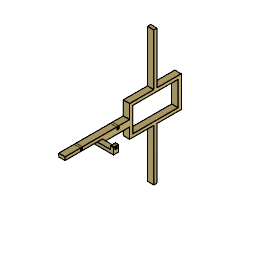
Cadru_Culisant (Autodesk Fusion 360 design; units mm, degrees)
part number: 2026-06-01-23-46-25-790
Autodesk Fusion 360 part; units mm, degrees
sketch "cadru" plane through (0, 0, 0) normal (1, 0, 0) x (0, 1, 0)
  line L0 (-20, -13.4697) -> (-20, 10.5303)
  line L1 (-17.5, -10.9697) -> (-17.5, 8.0303)
  line L2 (17.5, -10.9697) -> (-17.5, -10.9697)
  line L3 (20, -13.4697) -> (-20, -13.4697)
  line L4 (17.5, 8.0303) -> (17.5, -10.9697)
  line L5 (20, 10.5303) -> (20, -13.4697)
  line L6 (-20, 10.5303) -> (20, 10.5303)
  line L7 (-17.5, 8.0303) -> (17.5, 8.0303)
  line L8 (-1.25, 10.5303) -> (-1.25, 50.5303)
  line L9 (0, 0) -> (0, 50) construction
  line L10 (1.25, 10.5303) -> (1.25, 50.5303)
  line L11 (-1.25, 50.5303) -> (1.25, 50.5303)
  line L12 (17.5, -1.4697) -> (0, -1.4697) construction
  line L13 (-1.25, -53.4697) -> (1.25, -53.4697)
  line L14 (-1.25, -13.4697) -> (-1.25, -53.4697)
  line L15 (1.25, -13.4697) -> (1.25, -53.4697)
  line L16 (-20, -0.2197) -> (-70, -0.2197)
  line L17 (-70, -0.2197) -> (-70, -2.7197)
  line L18 (-70, -2.7197) -> (-20, -2.7197)
  line L19 (0, -1.4697) -> (-28.916, -1.4697) construction
  line L20 (-28.916, -1.4697) -> (-57.085, -1.4697) construction
  line L21 (-56.31, -0.6947) -> (-57.86, -0.6947)
  line L22 (-57.86, -0.6947) -> (-57.86, -2.2447)
  line L23 (-57.86, -2.2447) -> (-56.31, -2.2447)
  line L24 (-56.31, -2.2447) -> (-56.31, -0.6947)
  line L25 (-56.31, -0.6947) -> (-57.86, -2.2447) construction
  line L26 (-57.86, -0.6947) -> (-56.31, -2.2447) construction
  line L27 (-43.0005, -1.4697) -> (-43.0005, -15) construction
  line L28 (-45.0005, -5.2197) -> (-20, -5.2197)
  line L29 (-45.0005, -5.2197) -> (-45.0005, -0.2197)
  line L30 (-41.0005, -0.2197) -> (-41.0005, -5.2197)
  line L31 (-42.2255, -0.6947) -> (-43.7755, -0.6947)
  line L32 (-43.7755, -0.6947) -> (-43.7755, -2.2447)
  line L33 (-43.7755, -2.2447) -> (-42.2255, -2.2447)
  line L34 (-42.2255, -2.2447) -> (-42.2255, -0.6947)
  line L35 (-42.2255, -0.6947) -> (-43.7755, -2.2447) construction
  line L36 (-43.7755, -0.6947) -> (-42.2255, -2.2447) construction
  line L37 (-28.141, -0.6947) -> (-29.691, -0.6947)
  line L38 (-29.691, -0.6947) -> (-29.691, -2.2447)
  line L39 (-29.691, -2.2447) -> (-28.141, -2.2447)
  line L40 (-28.141, -2.2447) -> (-28.141, -0.6947)
  line L41 (-28.141, -0.6947) -> (-29.691, -2.2447) construction
  line L42 (-29.691, -0.6947) -> (-28.141, -2.2447) construction
  point P0 (-57.085, -1.4697)
  point P1 (-43.0005, -1.4697)
  point P2 (-28.916, -1.4697)
  dimension "d1" = -2.5
  dimension "d2" = 35
  dimension "d3" = 19
  dimension "d4" = 8.0303
  dimension "d5" = 17.5
  dimension "d6" = 40
  dimension "d7" = 1.25
  dimension "d10" = 50
  dimension "d11" = 2.5
  dimension "d12" = 1.25
  dimension "d13" = 28.916
  dimension "d15" = 28.169
  dimension "d16" = 1.55
  dimension "d17" = 1.55
  dimension "d22" = 14.0845
  dimension "d23" = 2.5
  dimension "d24" = 2
  dimension "d25" = 2
  dimension "d26" = 1.55
  dimension "d27" = 1.55
  dimension "d33" = 1.55
  dimension "d34" = 1.55
  constraint horizontal L7
  constraint vertical L4
  constraint horizontal L2
  constraint vertical L1
  constraint coincident L6 L8.start
  constraint perpendicular L6 L8
  constraint coincident L9.start origin
  constraint symmetric L8.start L9 L10.start
  constraint symmetric L8.end L9 L10.end
  constraint midpoint L4 L12.start
  constraint perpendicular L4 L12
  constraint symmetric L8.start L12 L14.start
  constraint symmetric L8.end L12 L13.start
  constraint symmetric L10.start L12 L15.start
  constraint symmetric L10.end L12 L13.end
  constraint coincident L0 L16.start
  constraint perpendicular L0 L16
  constraint perpendicular L16 L17
  constraint coincident L0 L18.end
  constraint perpendicular L0 L18
  constraint perpendicular L0 L19
  constraint parallel L19 L20
  constraint horizontal L21
  constraint perpendicular L21 L22
  constraint parallel L21 L23
  constraint parallel L22 L24
  constraint coincident L25 P0
  constraint coincident L26 P0
  constraint coincident P0 L20.end
  constraint coincident L20 P1
  constraint perpendicular L20 L27
  constraint coincident L0 L28.end
  constraint perpendicular L0 L28
  constraint coincident L16 L29.end
  constraint perpendicular L16 L29
  constraint coincident L16 L30.start
  constraint coincident L28 L30.end
  constraint perpendicular L28 L30
  constraint horizontal L31
  constraint perpendicular L31 L32
  constraint parallel L31 L33
  constraint parallel L32 L34
  constraint coincident L35 P1
  constraint coincident L36 P1
  constraint coincident P1 L27.start
  constraint horizontal L37
  constraint perpendicular L37 L38
  constraint parallel L37 L39
  constraint parallel L38 L40
  constraint coincident L41 P2
  constraint coincident L42 P2
  constraint coincident P2 L19.end
  measures "d2" distance of L4.start L1.end
  measures "d3" distance of L1.end L1.start
  measures "d4" distance of L9.start L7
  measures "d5" distance of L9.start L1
  measures "d6" distance of L8.start L8.end
  measures "d7" distance of L8 L9
  measures "d10" distance of L16.start L16.end
  measures "d11" distance of L16.end L17.end
  measures "d12" distance of L12 L16
  measures "d13" distance of L12.end P2
  measures "d15" distance of P2 P0
  measures "d16" distance of L22.end L23.end
  measures "d17" distance of L21.end L22.end
  measures "d22" distance of P0 L27
  measures "d23" distance of L18 L28
  measures "d24" distance of L27 L29
  measures "d25" distance of L27 L30
  measures "d26" distance of L32.end L33.end
  measures "d27" distance of L31.end L32.end
  measures "d33" distance of L38.end L39.end
  measures "d34" distance of L37.end L38.end
extrude "Extrude1" add sketch "cadru" along normal blind 5 contours L0 L3 L5 L6 | L0 L18 L28 L30 | L3 L13 L14 L15 | L0 L16 L18 L30 | L16 L18 L29 L30 | L16 L17 L18 L29 | L6 L8 L10 L11 | L31 L32 L33 L34
extrude "Extrude2" add sketch "cadru" along normal blind 15 contours L18 L28 L29 L30
extrude "Extrude3" add sketch "cadru" along normal blind 2.5 from surface at 15 contours L18 L28 L29 L30 | L16 L18 L29 L30
equation "d22 = ( 28.169 / 2 ) * 1 mm"
named bodies: "Cadru culisant"
